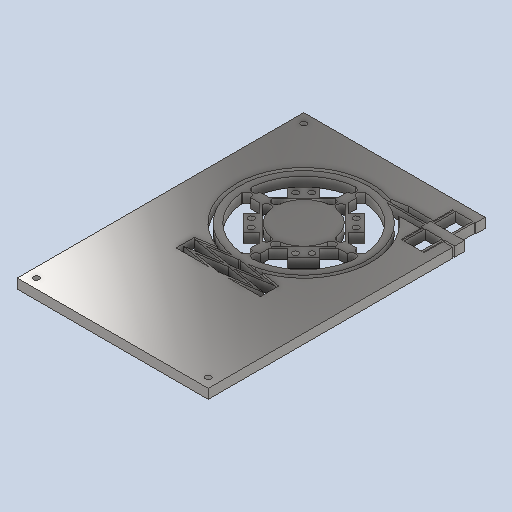
# Autodesk Inventor part: FlexBloc
Saved by Autodesk Inventor 2023 (Build 270158000, 158)
## iProperties
Created: 2023-03-17
Part Number: FlexBloc
Material: Steel, Mild
Document SubType Name: Modeling
Designer: Nathann
Density: 7.85 g/cm^3
Appearance: Semi-Polished
Mass: 505.648 g
Surface Area: 323.574 cm^2
Volume: 64.4137 cm^3
Author: Nathann
Autodesk Inventor part; units mm, degrees
ref_plane "YZ Plane" through (0, 0, 0) normal (1, 0, 0) x (0, 1, 0)
ref_plane "XZ Plane" through (0, 0, 0) normal (0, 1, 0) x (-1, 0, 0)
ref_plane "XY Plane" through (0, 0, 0) normal (0, 0, 1) x (1, 0, 0)
sketch "Sketch1" plane through (0, 0, 0) normal (0, 1, 0) x (-1, 0, 0)
  line L0 (0, 0) -> (100, 0)
  line L1 (100, 0) -> (100, 150)
  line L2 (100, 150) -> (0, 150)
  line L3 (0, 150) -> (0, 0)
  dimension "d0" = 150
  dimension "d1" = 100
  constraints: 8 end point, 2 parallel, 1 horizontal, 1 perpendicular
  measures "d0" distance of L2.end L0.start
  measures "d1" distance of L0.start L0.end
extrude "Extrusion1" add sketch "Sketch1" along normal blind 5
sketch "Sketch6" plane through (0, 5, 0) normal (0, 1, 0) x (1, 0, 0)
  circle A0 centre (-50, -50) radius 15
  line L0 (0, -150) -> (0, 0) projected
  line L1 (0, 0) -> (-100, 0) projected
  circle A1 centre (-50, -50) radius 30
  circle A2 centre (-50, -50) radius 33.541
  line L2 (-64.4545, -50.5) -> (-85.4944, -50.5)
  line L3 (-85.4944, -50.5) -> (-85.4944, -49.5)
  line L4 (-85.4944, -49.5) -> (-64.4545, -49.5)
  line L5 (-64.4545, -49.5) -> (-64.4545, -50.5)
  line L6 (-50, -50) -> (-59.276, -50)
  circle A3 centre (-50, -50) radius 36.041
  line L7 (-65, -50) -> (-80, -50)
  line L8 (-67.5, -50) -> (-70, -52.5)
  line L9 (-67.5, -50) -> (-70, -47.5)
  line L10 (-70, -52.5) -> (-70.7463, -51.7537)
  line L11 (-70, -47.5) -> (-74.2837, -51.7837)
  line L12 (-70, -52.5) -> (-72.5, -50)
  line L13 (-72.5, -50) -> (-70, -47.5)
  line L14 (-73.2071, -50) -> (-70.3536, -52.8536)
  line L15 (-70.3536, -52.8536) -> (-70, -52.5)
  line L16 (-73.2071, -50) -> (-70.3536, -47.1464)
  line L17 (-70.3536, -47.1464) -> (-70, -47.5)
  line L18 (-70.3536, -52.8536) -> (-65.8462, -57.3609)
  line L19 (-65.8462, -57.3609) -> (-65.1391, -56.6538)
  line L20 (-65.1391, -56.6538) -> (-69.6464, -52.1464)
  line L21 (-70.3536, -47.1464) -> (-65.8462, -42.6391)
  line L22 (-65.8462, -42.6391) -> (-65.1391, -43.3462)
  line L23 (-65.1391, -43.3462) -> (-69.6464, -47.8536)
  line L24 (-50, -50) -> (-54.8166, -54.8166)
  line L25 (-50, -50) -> (-57.7269, -42.2731)
  line L26 (-65.1391, -56.6538) -> (-70.0888, -61.6036)
  line L27 (-70.0888, -61.6036) -> (-65.8462, -65.8462)
  line L28 (-65.8462, -65.8462) -> (-60.8964, -60.8964)
  line L29 (-60.8964, -60.8964) -> (-65.1391, -56.6538)
  circle A4 centre (-65.8462, -61.6036) radius 1.5
  line L30 (-64.4545, -50) -> (-69.6304, -50)
  line L31 (-65.1391, -43.3462) -> (-70.0888, -38.3964)
  line L32 (-70.0888, -38.3964) -> (-65.8462, -34.1538)
  line L33 (-65.8462, -34.1538) -> (-60.8964, -39.1036)
  line L34 (-60.8964, -39.1036) -> (-65.1391, -43.3462)
  circle A5 centre (-65.8462, -38.3964) radius 1.5
  line L35 (-50, -64.4545) -> (-50, -69.6304)
  line L36 (-34.1538, -65.8462) -> (-39.1036, -60.8964)
  line L37 (-39.1036, -60.8964) -> (-43.3462, -65.1391)
  line L38 (-42.6391, -65.8462) -> (-43.3462, -65.1391)
  circle A6 centre (-38.3964, -65.8462) radius 1.5
  line L39 (-43.3462, -65.1391) -> (-38.3964, -70.0888)
  line L40 (-50, -67.5) -> (-52.5, -70)
  line L41 (-50, -67.5) -> (-47.5, -70)
  line L42 (-47.1464, -70.3536) -> (-42.6391, -65.8462)
  line L43 (-49.5, -64.4545) -> (-49.5, -85.4944)
  line L44 (-43.3462, -65.1391) -> (-47.8536, -69.6464)
  line L45 (-50.5, -85.4944) -> (-50.5, -64.4545)
  line L46 (-47.5, -70) -> (-48.2463, -70.7463)
  line L47 (-49.5, -85.4944) -> (-50.5, -85.4944)
  line L48 (-38.3964, -70.0888) -> (-34.1538, -65.8462)
  line L49 (-50.5, -64.4545) -> (-49.5, -64.4545)
  line L50 (-50, -65) -> (-50, -80)
  line L51 (-47.1464, -70.3536) -> (-47.5, -70)
  line L52 (-52.8536, -70.3536) -> (-52.5, -70)
  line L53 (-47.5, -70) -> (-50, -72.5)
  line L54 (-50, -73.2071) -> (-47.1464, -70.3536)
  line L55 (-50, -72.5) -> (-52.5, -70)
  line L56 (-50, -73.2071) -> (-52.8536, -70.3536)
  line L57 (-52.5, -70) -> (-48.2163, -74.2837)
  line L58 (-56.6538, -65.1391) -> (-52.1464, -69.6464)
  line L59 (-52.8536, -70.3536) -> (-57.3609, -65.8462)
  line L60 (-60.8964, -60.8964) -> (-56.6538, -65.1391)
  line L61 (-56.6538, -65.1391) -> (-61.6036, -70.0888)
  circle A7 centre (-61.6036, -65.8462) radius 1.5
  line L62 (-65.8462, -65.8462) -> (-60.8964, -60.8964)
  line L63 (-61.6036, -70.0888) -> (-65.8462, -65.8462)
  line L64 (-57.3609, -65.8462) -> (-56.6538, -65.1391)
  line L65 (-35.5455, -50) -> (-30.3696, -50)
  line L66 (-34.1538, -34.1538) -> (-39.1036, -39.1036)
  line L67 (-39.1036, -39.1036) -> (-34.8609, -43.3462)
  line L68 (-34.1538, -42.6391) -> (-34.8609, -43.3462)
  circle A8 centre (-34.1538, -38.3964) radius 1.5
  line L69 (-34.8609, -43.3462) -> (-29.9112, -38.3964)
  line L70 (-32.5, -50) -> (-30, -52.5)
  line L71 (-32.5, -50) -> (-30, -47.5)
  line L72 (-29.6464, -47.1464) -> (-34.1538, -42.6391)
  line L73 (-35.5455, -49.5) -> (-14.5056, -49.5)
  line L74 (-34.8609, -43.3462) -> (-30.3536, -47.8536)
  line L75 (-14.5056, -50.5) -> (-35.5455, -50.5)
  line L76 (-30, -47.5) -> (-29.2537, -48.2463)
  line L77 (-14.5056, -49.5) -> (-14.5056, -50.5)
  line L78 (-29.9112, -38.3964) -> (-34.1538, -34.1538)
  line L79 (-35.5455, -50.5) -> (-35.5455, -49.5)
  line L80 (-35, -50) -> (-20, -50)
  line L81 (-29.6464, -47.1464) -> (-30, -47.5)
  line L82 (-29.6464, -52.8536) -> (-30, -52.5)
  line L83 (-30, -47.5) -> (-27.5, -50)
  line L84 (-26.7929, -50) -> (-29.6464, -47.1464)
  line L85 (-27.5, -50) -> (-30, -52.5)
  line L86 (-26.7929, -50) -> (-29.6464, -52.8536)
  line L87 (-30, -52.5) -> (-25.7163, -48.2163)
  line L88 (-34.8609, -56.6538) -> (-30.3536, -52.1464)
  line L89 (-29.6464, -52.8536) -> (-34.1538, -57.3609)
  line L90 (-39.1036, -60.8964) -> (-34.8609, -56.6538)
  line L91 (-34.8609, -56.6538) -> (-29.9112, -61.6036)
  circle A9 centre (-34.1538, -61.6036) radius 1.5
  line L92 (-34.1538, -65.8462) -> (-39.1036, -60.8964)
  line L93 (-29.9112, -61.6036) -> (-34.1538, -65.8462)
  line L94 (-34.1538, -57.3609) -> (-34.8609, -56.6538)
  line L95 (-50, -35.5455) -> (-50, -30.3696)
  line L96 (-65.8462, -34.1538) -> (-60.8964, -39.1036)
  line L97 (-60.8964, -39.1036) -> (-56.6538, -34.8609)
  line L98 (-57.3609, -34.1538) -> (-56.6538, -34.8609)
  circle A10 centre (-61.6036, -34.1538) radius 1.5
  line L99 (-56.6538, -34.8609) -> (-61.6036, -29.9112)
  line L100 (-50, -32.5) -> (-47.5, -30)
  line L101 (-50, -32.5) -> (-52.5, -30)
  line L102 (-52.8536, -29.6464) -> (-57.3609, -34.1538)
  line L103 (-50.5, -35.5455) -> (-50.5, -14.5056)
  line L104 (-56.6538, -34.8609) -> (-52.1464, -30.3536)
  line L105 (-49.5, -14.5056) -> (-49.5, -35.5455)
  line L106 (-52.5, -30) -> (-51.7537, -29.2537)
  line L107 (-50.5, -14.5056) -> (-49.5, -14.5056)
  line L108 (-61.6036, -29.9112) -> (-65.8462, -34.1538)
  line L109 (-49.5, -35.5455) -> (-50.5, -35.5455)
  line L110 (-50, -35) -> (-50, -20)
  line L111 (-52.8536, -29.6464) -> (-52.5, -30)
  line L112 (-47.1464, -29.6464) -> (-47.5, -30)
  line L113 (-52.5, -30) -> (-50, -27.5)
  line L114 (-50, -26.7929) -> (-52.8536, -29.6464)
  line L115 (-50, -27.5) -> (-47.5, -30)
  line L116 (-50, -26.7929) -> (-47.1464, -29.6464)
  line L117 (-47.5, -30) -> (-51.7837, -25.7163)
  line L118 (-43.3462, -34.8609) -> (-47.8536, -30.3536)
  line L119 (-47.1464, -29.6464) -> (-42.6391, -34.1538)
  line L120 (-39.1036, -39.1036) -> (-43.3462, -34.8609)
  line L121 (-43.3462, -34.8609) -> (-38.3964, -29.9112)
  circle A11 centre (-38.3964, -34.1538) radius 1.5
  line L122 (-34.1538, -34.1538) -> (-39.1036, -39.1036)
  line L123 (-38.3964, -29.9112) -> (-34.1538, -34.1538)
  line L124 (-42.6391, -34.1538) -> (-43.3462, -34.8609)
  point P0 (-67.9675, -36.2751)
  point P1 (-63.7249, -67.9675)
  point P2 (-32.0325, -63.7249)
  point P3 (-36.2751, -32.0325)
  point P4 (-49.5, -72.7071)
  point P5 (-49.5, -79.9958)
  point P6 (-20.0042, -50.5)
  point P7 (-27.2929, -50.5)
  point P8 (-34.1538, -42.6391)
  point P9 (-27.2929, -49.5)
  point P10 (-20.0042, -49.5)
  point P11 (-49.5, -20.0042)
  point P12 (-49.5, -27.2929)
  point P13 (-68, -49.5)
  point P14 (-64.9917, -49.5)
  point P15 (-50.5, -35.0083)
  point P16 (-50.5, -32)
  point P17 (-49.5, -32)
  point P18 (-49.5, -35.0083)
  point P19 (-35.0083, -49.5)
  point P20 (-32, -49.5)
  point P21 (-32, -50.5)
  point P22 (-35.0083, -50.5)
  point P23 (-49.5, -64.9917)
  point P24 (-49.5, -68)
  point P25 (-50.5, -68)
  point P26 (-50.5, -64.9917)
  point P27 (-64.9917, -50.5)
  point P28 (-68, -50.5)
  point P29 (-57.3609, -34.1538)
  point P30 (-50.5, -27.2929)
  point P31 (-50.5, -20.0042)
  point P32 (-79.9958, -49.5)
  point P33 (-72.7071, -49.5)
  point P34 (-72.7071, -50.5)
  point P35 (-79.9958, -50.5)
  point P36 (-50.5, -79.9958)
  point P37 (-50.5, -72.7071)
  point P38 (-83.5373, -50.5)
  point P39 (-83.5373, -49.5)
  point P40 (-50.5, -16.4627)
  point P41 (-49.5, -16.4627)
  point P42 (-16.4627, -49.5)
  point P43 (-16.4627, -50.5)
  point P44 (-49.5, -83.5373)
  point P45 (-50.5, -83.5373)
  dimension "d80" = 30
  dimension "d81" = 60
  dimension "d78" = 50
  dimension "d79" = 50
  dimension "d82" = 67.082
  dimension "d83" = 0.5
  dimension "d84" = 0.5
  dimension "d91" = 72.082
  dimension "d92" = 5
  dimension "d93" = 2.5
  dimension "d94" = 2.5
  dimension "d95" = 45
  dimension "d96" = 45
  dimension "d97" = 0.5
  dimension "d98" = 0.5
  dimension "d99" = 0.5
  dimension "d100" = 45
  dimension "d101" = 45
  dimension "d102" = 6
  dimension "d103" = 7
  dimension "d104" = 3
  dimension "d105" = 3
  dimension "d106" = 3
  dimension "d107" = 3
  dimension "d108" = 7.5
  dimension "d109" = 3
  dimension "d110" = 6
  dimension "d111" = 7
  dimension "d112" = 3
  dimension "d113" = 3
  dimension "d114" = 3
  dimension "d117" = 360
  constraints: 246 end point, 20 point on line, 15 perpendicular, 10 centre point, 9 parallel, 3 coincident, 3 horizontal, 3 midpoint, 264 other
  measures "d78" distance from line of point (-50, -50) L0
  measures "d79" distance from line of L1 point (-50, -50)
  measures "d82" diameter of A2
  measures "d83" distance between parallel lines of L4 L6
  measures "d84" distance from line of point (-50, -50) L2
  measures "d91" diameter of A3
  measures "d92" distance of L8.start L12.end
  measures "d93" horizontal distance of L12.end L9.end
  measures "d94" horizontal distance of L8.end L12.end
  measures "d95" angle of L7 L8
  measures "d96" angle of L9 L7
  measures "d97" distance of L14.end L8.end
  measures "d98" distance between parallel lines of L10 L20
  measures "d99" distance between parallel lines of L23 L11
  measures "d100" angle of L24 L6
  measures "d101" angle of L25 L6
  measures "d102" distance of L28.end L19.end
  measures "d103" distance of L19.end L26.end
  measures "d104" distance from line of L27 A4.centre
  measures "d105" distance from line of L26 A4.centre
  measures "d106" diameter of A4
  measures "d107" distance from line of L24 A4.centre
  measures "d108" distance of L7.start L12.end
  measures "d109" distance of point (-67.968, -36.275) A5.centre
  measures "d110" distance of L33.end L22.end
  measures "d111" distance of L32.end L33.end
  measures "d112" distance from line of L33 A5.centre
  measures "d113" diameter of A5
  measures "d114" distance from line of A5.centre L25
extrude "Extrusion6" cut sketch "Sketch6" against normal blind 10 contours A0 L105 L100 L118 L120 L67 L74 L71 L73 | L75 L70 L88 L90 L37 L44 L41 L43 A0 | A0 L4 L9 L23 L34 L97 L104 L101 L103 | L84 L72 L69 L78 L123 L121 L119 L116 L105 A1 L73 | L45 L40 L58 L60 L29 L20 L8 L2 A0 | L75 A1 L43 L54 L42 L39 L48 L93 L91 L89 L86 | A2 L73 L77 L75 | L114 L102 L99 L108 L32 L31 L21 L16 L4 A1 L103 | A2 L103 L107 L105 | L45 A1 L2 L14 L18 L26 L27 L63 L61 L59 L56 | L43 L47 L45 A2 | A2 L2 L3 L4 | A4 | A5 | A6 | A7 | A8 | A9 | A10 | A11
sketch "Sketch7" plane through (0, 5, 0) normal (0, 1, 0) x (1, 0, 0)
  line L0 (-30.2515, -22) -> (6.5047, -22)
  line L1 (6.5047, -22) -> (6.5047, -15)
  line L2 (6.5047, -15) -> (-23.9617, -15)
  line L3 (-50, -60) -> (-28.7023, -38.7023)
  line L4 (-50, -60) -> (0, -60)
  line L5 (-11.682, -22) -> (-5.682, -22)
  line L6 (-2.365, -15) -> (-8.365, -15)
  line L7 (-5, -22) -> (-17, -22)
  line L8 (-17, -22) -> (-17, -32)
  line L9 (-17, -32) -> (-5, -32)
  line L10 (-5, -32) -> (-5, -22)
  line L11 (-5, -15) -> (-17, -15)
  line L12 (-17, -15) -> (-17, -5)
  line L13 (-17, -5) -> (-5, -5)
  line L14 (-5, -5) -> (-5, -15)
  line L15 (0, 0) -> (-100, 0) projected
  line L16 (0, -150) -> (0, 0) projected
  line L17 (-16.5, -32) -> (-15.5, -32)
  line L18 (-15.5, -32) -> (-15.5, -21)
  line L19 (-15.5, -21) -> (-16.5, -21)
  line L20 (-16.5, -21) -> (-16.5, -32)
  line L21 (-5.5, -32) -> (-6.5, -32)
  line L22 (-6.5, -32) -> (-6.5, -21)
  line L23 (-6.5, -21) -> (-5.5, -21)
  line L24 (-5.5, -21) -> (-5.5, -32)
  line L25 (-5.5, -5) -> (-6.5, -5)
  line L26 (-6.5, -5) -> (-6.5, -16)
  line L27 (-6.5, -16) -> (-5.5, -16)
  line L28 (-5.5, -16) -> (-5.5, -5)
  line L29 (-16.5, -5) -> (-15.5, -5)
  line L30 (-15.5, -5) -> (-15.5, -16)
  line L31 (-15.5, -16) -> (-16.5, -16)
  line L32 (-16.5, -16) -> (-16.5, -5)
  line L33 (-17.539, -21) -> (0, -21)
  line L34 (0, -21) -> (0, -16)
  line L35 (0, -16) -> (-17.539, -16)
  arc A0 (-49.5, -16.4627) -> (-50.5, -16.4627) centre (-50, -50) ccw projected
  line L36 (0, 0) -> (-5, 0)
  line L37 (-5, 0) -> (-5, -16)
  line L38 (-5, -16) -> (0, -16)
  line L39 (0, -16) -> (0, 0)
  line L40 (-17.539, -21) -> (-17.539, -16)
  line L41 (-20.9617, -19) -> (-17.539, -19)
  line L42 (-17.539, -19) -> (-17.539, -18)
  line L43 (-17.539, -18) -> (-20.9617, -18)
  line L44 (-23.9617, -15) -> (-23.9617, -22)
  line L45 (-23.9617, -22) -> (-30.2515, -22)
  line L46 (-20.9617, -18) -> (-20.9617, -19)
  point P0 (-5.5, -10.5)
  point P1 (-5, -27)
  point P2 (-16, -21)
  point P3 (-16, -16)
  point P4 (-17, -15)
  point P5 (-17, -22)
  point P6 (-15.5, -5)
  point P7 (-15.5, -16)
  point P8 (-6.5, -16)
  point P9 (-6.5, -5)
  point P10 (-5.5, -16)
  point P11 (0, -16)
  point P12 (0, -15)
  point P13 (0, -21)
  point P14 (0, -22)
  point P15 (-6.5, -32)
  point P16 (-5, -5)
  point P17 (-15.5, -15)
  point P18 (-16.5, -15)
  point P19 (-15.5, -22)
  point P20 (-16.5, -22)
  point P21 (-16.5, -15)
  point P22 (-16.5, -22)
  point P23 (-6.5, -22)
  point P24 (-15.5, -22)
  point P25 (-5.5, -22)
  point P26 (-5.5, -15)
  point P27 (-15.5, -15)
  point P28 (-6.5, -15)
  dimension "d125" = 45
  dimension "d128" = 10
  dimension "d133" = 12
  dimension "d134" = 12
  dimension "d135" = 5
  dimension "d136" = 1
  dimension "d137" = 1
  dimension "d138" = 1
  dimension "d139" = 1
  dimension "d140" = 0.5
  dimension "d141" = 0.5
  dimension "d142" = 11
  dimension "d144" = 11
  dimension "d145" = 11
  dimension "d146" = 10
  dimension "d147" = 11
  dimension "d164" = 5
  dimension "d169" = 0
  dimension "d170" = 5
  dimension "d171" = 1
  dimension "d172" = 2
  dimension "d202" = 5
  dimension "d214" = 3
  constraints: 90 end point, 17 parallel, 17 point on line, 13 horizontal, 12 perpendicular, 4 midpoint, 2 vertical
  measures "d125" angle of L3 L4
  measures "d128" distance of L9.end L7.start
  measures "d133" distance of L8.end L9.end
  measures "d134" distance of L12.end L13.end
  measures "d135" distance between parallel lines of L16 L10
  measures "d136" distance between parallel lines of L18 L20
  measures "d137" distance between parallel lines of L22 L24
  measures "d138" distance from line of L26 point (-5.5, -10.5)
  measures "d139" distance between parallel lines of L32 L30
  measures "d140" distance between parallel lines of L8 L20
  measures "d141" distance from line of point (-5, -27) L24
  measures "d142" distance of L17.end L18.end
  measures "d144" distance of L29.end L30.end
  measures "d145" distance of L27.end L25.start
  measures "d146" distance of L11.end L12.end
  measures "d147" distance of L21.end L22.end
  measures "d164" distance between parallel lines of L16 L37
  measures "d169" distance between parallel lines of L34 L16
  measures "d170" distance between parallel lines of L35 L33
  measures "d171" distance between parallel lines of L43 L41
  measures "d172" distance between parallel lines of L35 L43
  measures "d202" distance between parallel lines of L15 L13
  measures "d214" distance between parallel lines of L46 L44
extrude "Extrusion7" cut sketch "Sketch7" against normal blind 5 contours L44 L2 L32 L35 L40 L43 L46 L41 L33 L20 L0 | L0 L20 L9 L8 | L12 L13 L32 L2 | L18 L33 L22 L0 | L0 L22 L9 L18 | L30 L13 L26 L2 | L2 L26 L35 L30 | L24 L0 L10 L9 | L33 L16 L0 L24 | L16 L2 L1 L0 | L28 L13 L14 L2 | L2 L37 L35 L28 | L35 L37 L2 L16 | L14 L37 L15 L16 L2
sketch "Sketch9" plane through (0, 5, 0) normal (0, 1, 0) x (1, 0, 0)
  arc A0 (-35.0083, -49.5) -> (-49.5, -35.0083) centre (-50, -50) ccw projected
  line L0 (-50, -50) -> (-50, -7.3451)
  arc A1 (-49.5, -16.4627) -> (-50.5, -16.4627) centre (-50, -50) ccw projected
  line L1 (-50, -16.459) -> (-35, -13.959)
  line L2 (-35, -13.959) -> (-50, -11.459)
  line L3 (-50, -11.459) -> (-65, -13.959)
  line L4 (-65, -13.959) -> (-50, -16.459)
  line L5 (-50, -17.4728) -> (-28.9172, -13.959)
  line L6 (-28.9172, -13.959) -> (-50, -10.4452)
  line L7 (-50, -10.4452) -> (-71.0828, -13.959)
  line L8 (-71.0828, -13.959) -> (-50, -17.4728)
  line L9 (-28.9172, -13.959) -> (-71.0828, -13.959)
  line L10 (-65, -7.9452) -> (-50, -10.4452)
  line L11 (-71.0828, -7.9452) -> (-50, -11.459)
  line L12 (-50, -5.4452) -> (-65, -7.9452)
  line L13 (-50, -4.4314) -> (-71.0828, -7.9452)
  line L14 (-28.9172, -7.9452) -> (-71.0828, -7.9452)
  line L15 (-35, -7.9452) -> (-50, -5.4452)
  line L16 (-50, -11.459) -> (-28.9172, -7.9452)
  line L17 (-28.9172, -7.9452) -> (-50, -4.4314)
  line L18 (-50, -10.4452) -> (-35, -7.9452)
  arc A2 (-49.5, -16.4627) -> (-50.5, -16.4627) centre (-50, -50) ccw projected
  line L19 (-50, -50) -> (-50, -44.5788)
  line L20 (-57.3177, -17.267) -> (-72.0828, -14.8061)
  line L21 (-72.0828, -14.8061) -> (-72.0828, -5.2647)
  line L22 (-42.6823, -17.267) -> (-27.9172, -14.8061)
  line L23 (-27.9172, -14.8061) -> (-27.9172, -5.2647)
  line L24 (-23.9617, -15) -> (-17, -15) projected
  line L25 (-27.9172, -5.2647) -> (-45, -5.2647)
  line L26 (-55, -5.2647) -> (-72.0828, -5.2647)
  line L27 (-57.3177, -17.267) -> (-54.3685, -16.7447)
  line L28 (-42.6823, -17.267) -> (-45.6315, -16.7447)
  line L29 (-57.3177, -50) -> (-38.2747, -50)
  line L30 (-50, -83.541) -> (-35, -86.041)
  line L31 (-35, -86.041) -> (-50, -88.541)
  line L32 (-50, -88.541) -> (-65, -86.041)
  line L33 (-65, -86.041) -> (-50, -83.541)
  line L34 (-50, -82.5272) -> (-28.9172, -86.041)
  line L35 (-28.9172, -86.041) -> (-50, -89.5548)
  line L36 (-50, -89.5548) -> (-71.0828, -86.041)
  line L37 (-71.0828, -86.041) -> (-50, -82.5272)
  line L38 (-28.9172, -86.041) -> (-71.0828, -86.041)
  line L39 (-65, -92.0548) -> (-50, -89.5548)
  line L40 (-71.0828, -92.0548) -> (-50, -88.541)
  line L41 (-50, -94.5548) -> (-65, -92.0548)
  line L42 (-50, -95.5686) -> (-71.0828, -92.0548)
  line L43 (-28.9172, -92.0548) -> (-71.0828, -92.0548)
  line L44 (-35, -92.0548) -> (-50, -94.5548)
  line L45 (-50, -88.541) -> (-28.9172, -92.0548)
  line L46 (-28.9172, -92.0548) -> (-50, -95.5686)
  line L47 (-50, -89.5548) -> (-35, -92.0548)
  line L48 (-57.3177, -82.733) -> (-72.0828, -85.1939)
  line L49 (-72.0828, -85.1939) -> (-72.0828, -94.7353)
  line L50 (-42.6823, -82.733) -> (-27.9172, -85.1939)
  line L51 (-27.9172, -85.1939) -> (-27.9172, -94.7353)
  line L52 (-27.9172, -94.7353) -> (-45, -94.7353)
  line L53 (-55, -94.7353) -> (-72.0828, -94.7353)
  line L54 (-57.3177, -82.733) -> (-54.3685, -83.2553)
  line L55 (-42.6823, -82.733) -> (-45.6315, -83.2553)
  point P0 (0, 0)
  point P1 (-16.459, -50)
  point P2 (-16.459, -50)
  point P3 (-50, -1.3313)
  point P4 (-51, -4.2647)
  point P5 (-51, -4.5981)
  point P6 (-53.0414, -10.9521)
  point P7 (-46.9586, -10.9521)
  point P8 (-45.6315, -16.7447)
  point P9 (-51.4257, -26.4893)
  point P10 (-50, -26.459)
  point P11 (-42.6823, -17.267)
  point P12 (-57.3177, -17.267)
  point P13 (-49.5, -64.9917)
  point P14 (-50, -92.6549)
  point P15 (-50, -98.6687)
  point P16 (-51, -95.7353)
  point P17 (-51, -95.4019)
  point P18 (-51.4257, -73.5107)
  point P19 (-50, -73.541)
  point P20 (-50, -55.4212)
  point P21 (-23.9617, -85)
  point P22 (-49.5, -83.5373)
  point P23 (-50.5, -83.5373)
  point P24 (-53.0414, -89.0479)
  point P25 (-46.9586, -89.0479)
  dimension "d167" = 5
  dimension "d168" = 1
  dimension "d179" = 1
  dimension "d180" = 1
  dimension "d182" = 1.0138
  dimension "d185" = 6.0138
  dimension "d190" = 1
  dimension "d191" = 1
  dimension "d203" = 0
  dimension "d204" = 1
  dimension "d205" = 1
  dimension "d206" = 1
  dimension "d207" = 1
  dimension "d208" = 5
  dimension "d209" = 5
  constraints: 110 end point, 37 symmetric about line, 19 point on line, 5 equal length, 5 parallel, 4 horizontal, 3 vertical, 2 perpendicular, 34 other
  measures "d167" distance of L1.start L2.end
  measures "d168" distance between parallel lines of L5 L1
  measures "d179" distance between parallel lines of L8 L4
  measures "d180" distance between parallel lines of L7 L3
  measures "d182" distance of L5.start L1.start
  measures "d185" distance of L5.start L11.end
  measures "d190" horizontal distance of L13.start point (-51, -4.265)
  measures "d191" horizontal distance of point (-51, -4.598) L13.start
  measures "d203" distance between parallel lines of L19 L0
  measures "d204" distance between parallel lines of L8 L20
  measures "d205" distance between parallel lines of L5 L22
  measures "d206" distance from line of L5.end L23
  measures "d207" distance from line of L21 L7.end
  measures "d208" horizontal distance of L25.end L13.start
  measures "d209" horizontal distance of L13.start L26.start
extrude "Extrusion10" cut sketch "Sketch9" against normal blind 5 contours L30 L38 L33 | L31 L32 L38 | L34 L55 L50 L51 L52 L46 L45 L35 | L36 L40 L42 L53 L49 L48 L54 L37 | L47 L43 L39 | L43 L44 L41
sketch "Sketch11" plane through (0, 5, 0) normal (0, 1, 0) x (1, 0, 0)
  arc A0 (-64.9917, -50.5) -> (-50.5, -64.9917) centre (-50, -50) ccw projected
  circle A1 centre (-50, -50) radius 33.541
  line L0 (-49.5, -85.4944) -> (-49.5, -83.5373) projected
  arc A2 (-74.717, -75.4789) -> (-25.283, -75.4789) centre (-50, -50) ccw
  arc A3 (-15.5761, -58.6662) -> (-40.2932, -15.855) centre (-50, -50) ccw
  arc A4 (-59.7068, -15.855) -> (-84.8937, -56.5221) centre (-50, -50) ccw
  circle A5 centre (-50, -50) radius 35.498
  line L1 (-57.3177, -82.733) -> (-54.3685, -83.2553) projected
  line L2 (-57.3177, -82.733) -> (-61.7985, -83.4799)
  line L3 (-57.3177, -82.733) -> (-72.0828, -85.1939) projected
  line L4 (-27.9172, -85.1939) -> (-42.6823, -82.733) projected
  line L5 (-38.2015, -83.4799) -> (-42.6823, -82.733)
  point P0 (0, 0)
  point P1 (-82.0065, -60.0292)
  point P2 (-38.2015, -83.4799)
  point P3 (-25.283, -75.4789)
  point P4 (-40.2932, -15.855)
  point P5 (-59.7068, -15.855)
  dimension "d220" = 67.082
  constraints: 11 point on circle, 5 centre point, 4 end point, 3 coincident, 2 point on line, 1 collinear
  measures "d220" diameter of A1
extrude "Extrusion11" cut sketch "Sketch11" against normal blind 5 contours A1 L2 A2 A5 A4 A3 L4
sketch "Sketch12" plane through (0, 5, 0) normal (0, 1, 0) x (1, 0, 0)
  line L0 (-17, -15) -> (-23.9617, -15) projected
  line L1 (-23.9617, -15) -> (-30.0605, -15)
  line L2 (-30.0605, -15) -> (-30.0605, -22)
  line L3 (-30.0605, -22) -> (-23.9617, -22)
  line L4 (-23.9617, -22) -> (-23.9617, -15)
  line L5 (-30.0605, -22) -> (-38.2015, -16.5201)
  line L6 (-38.2015, -16.5201) -> (-30.0605, -15)
  point P0 (0, 0)
  constraints: 12 end point, 2 parallel, 1 horizontal, 1 perpendicular
extrude "Extrusion12" cut sketch "Sketch12" against normal blind 5
sketch "Sketch13" plane through (0, 5, 0) normal (0, 1, 0) x (1, 0, 0)
  line L0 (-17.539, -18) -> (-20.9617, -18) projected
  line L1 (-20.9617, -18) -> (-41.4723, -18)
  line L2 (-41.4723, -18) -> (-41.4723, -19)
  line L3 (-41.4723, -19) -> (-20.9617, -19)
  line L4 (-20.9617, -19) -> (-20.9617, -18)
  point P0 (0, 0)
  constraints: 8 end point, 2 parallel, 1 horizontal, 1 perpendicular
extrude "Extrusion13" add sketch "Sketch13" against normal blind 5
sketch "Sketch14" plane through (0, 5, 0) normal (0, 1, 0) x (1, 0, 0)
  circle A0 centre (-95, -5) radius 1.5
  circle A1 centre (-95, -145) radius 1.5
  circle A2 centre (-5, -145) radius 1.5
  line L0 (0, -150) -> (0, -22) projected
  line L1 (-100, -150) -> (0, -150) projected
  line L2 (-100, 0) -> (-100, -150) projected
  line L3 (-5, 0) -> (-100, 0) projected
  point P0 (0, 0)
  dimension "d227" = 5
  dimension "d228" = 5
  dimension "d229" = 5
  dimension "d230" = 5
  dimension "d231" = 5
  dimension "d232" = 5
  dimension "d233" = 3
  dimension "d234" = 3
  dimension "d235" = 3
  constraints: 3 centre point
  measures "d227" distance from line of L0 A2.centre
  measures "d228" distance from line of L1 A2.centre
  measures "d229" distance from line of L1 A1.centre
  measures "d230" distance from line of L2 A1.centre
  measures "d231" distance from line of L3 A0.centre
  measures "d232" distance from line of L2 A0.centre
  measures "d233" diameter of A0
  measures "d234" diameter of A1
  measures "d235" diameter of A2
extrude "Extrusion14" cut sketch "Sketch14" against normal blind 5
sketch "Sketch15" plane through (0, 5, 0) normal (0, 1, 0) x (1, 0, 0)
  line L0 (-47.5, -64.5161) -> (-52.5, -64.5161)
  line L1 (-52.5, -80.5042) -> (-47.5, -80.5042)
  arc A0 (-50.5, -35.0083) -> (-64.9917, -49.5) centre (-50, -50) ccw projected
  line L2 (-50, -50) -> (-45.827, -50)
  line L3 (-50.5, -72.7071) -> (-50.5, -79.9958) projected
  line L4 (-49.5, -68) -> (-49.5, -64.9917) projected
  circle A1 centre (-47.5, -77.5042) radius 2.15
  circle A2 centre (-52.5, -77.5042) radius 2.15
  line L5 (-50.5, -64.9917) -> (-50.5, -68) projected
  circle A3 centre (-52.5, -66.9902) radius 2.15
  circle A4 centre (-47.5, -66.9902) radius 2.15
  arc A5 (-79.9958, -50.5) -> (-50.5, -79.9958) centre (-50, -50) ccw projected
  line L6 (-50.5, -79.9958) -> (-49.5001, -80.0125)
  line L7 (-52.5, -64.7902) -> (-47.5, -64.7902)
  arc A6 (-49.5, -64.9917) -> (-35.0083, -50.5) centre (-50, -50) ccw projected
  line L8 (-52.5, -79.6542) -> (-52.5, -80.5042)
  line L9 (-47.5, -80.5042) -> (-47.5, -79.6542)
  line L10 (-47.5, -75.3542) -> (-47.5, -69.1402)
  line L11 (-47.5, -64.8402) -> (-47.5, -64.5161)
  line L12 (-52.5, -64.5161) -> (-52.5, -64.8402)
  line L13 (-52.5, -69.1402) -> (-52.5, -75.3542)
  circle A7 centre (-22.4958, -52.5) radius 2.15
  line L14 (-30.8598, -52.5) -> (-24.6458, -52.5)
  circle A8 centre (-33.0098, -52.5) radius 2.15
  line L15 (-35.4839, -47.5) -> (-35.4839, -52.5)
  line L16 (-35.1598, -47.5) -> (-35.4839, -47.5)
  line L17 (-35.4839, -52.5) -> (-35.1598, -52.5)
  circle A9 centre (-33.0098, -47.5) radius 2.15
  line L18 (-35.2098, -52.5) -> (-35.2098, -47.5)
  line L19 (-20.3458, -52.5) -> (-19.4958, -52.5)
  line L20 (-20.0042, -50.5) -> (-19.9875, -49.5001)
  line L21 (-24.6458, -47.5) -> (-30.8598, -47.5)
  line L22 (-19.4958, -52.5) -> (-19.4958, -47.5)
  line L23 (-19.4958, -47.5) -> (-20.3458, -47.5)
  circle A10 centre (-22.4958, -47.5) radius 2.15
  circle A11 centre (-47.5, -22.4958) radius 2.15
  line L24 (-47.5, -30.8598) -> (-47.5, -24.6458)
  circle A12 centre (-47.5, -33.0098) radius 2.15
  line L25 (-52.5, -35.4839) -> (-47.5, -35.4839)
  line L26 (-52.5, -35.1598) -> (-52.5, -35.4839)
  line L27 (-47.5, -35.4839) -> (-47.5, -35.1598)
  circle A13 centre (-52.5, -33.0098) radius 2.15
  line L28 (-47.5, -35.2098) -> (-52.5, -35.2098)
  line L29 (-47.5, -20.3458) -> (-47.5, -19.4958)
  line L30 (-49.5, -20.0042) -> (-50.4999, -19.9875)
  line L31 (-52.5, -24.6458) -> (-52.5, -30.8598)
  line L32 (-47.5, -19.4958) -> (-52.5, -19.4958)
  line L33 (-52.5, -19.4958) -> (-52.5, -20.3458)
  circle A14 centre (-52.5, -22.4958) radius 2.15
  circle A15 centre (-77.5042, -47.5) radius 2.15
  line L34 (-69.1402, -47.5) -> (-75.3542, -47.5)
  circle A16 centre (-66.9902, -47.5) radius 2.15
  line L35 (-64.5161, -52.5) -> (-64.5161, -47.5)
  line L36 (-64.8402, -52.5) -> (-64.5161, -52.5)
  line L37 (-64.5161, -47.5) -> (-64.8402, -47.5)
  circle A17 centre (-66.9902, -52.5) radius 2.15
  line L38 (-64.7902, -47.5) -> (-64.7902, -52.5)
  line L39 (-79.6542, -47.5) -> (-80.5042, -47.5)
  line L40 (-79.9958, -49.5) -> (-80.0125, -50.4999)
  line L41 (-75.3542, -52.5) -> (-69.1402, -52.5)
  line L42 (-80.5042, -47.5) -> (-80.5042, -52.5)
  line L43 (-80.5042, -52.5) -> (-79.6542, -52.5)
  circle A18 centre (-77.5042, -52.5) radius 2.15
  point P0 (0, 0)
  point P1 (-50.5, -66.4958)
  point P2 (-50, -80.5042)
  point P3 (-50.0001, -80.0042)
  point P4 (-33.5042, -50.5)
  point P5 (-19.9958, -50.0001)
  point P6 (-19.4958, -50)
  point P7 (-49.5, -33.5042)
  point P8 (-49.9999, -19.9958)
  point P9 (-50, -19.4958)
  point P10 (-66.4958, -49.5)
  point P11 (-80.0042, -49.9999)
  point P12 (-80.5042, -50)
  point P13 (-49.5, -66.2012)
  dimension "d238" = 2
  dimension "d240" = 0.7
  dimension "d241" = 4.3
  dimension "d243" = 1
  dimension "d244" = 3
  dimension "d245" = 3
  dimension "d246" = 0.5
  dimension "d247" = 4.3
  dimension "d248" = 4.3
  dimension "d249" = 2.2
  dimension "d250" = 2.2
  dimension "d253" = 360
  constraints: 82 end point, 33 point on circle, 16 centre point, 10 parallel, 8 point on line, 3 midpoint, 3 perpendicular, 2 horizontal, 1 tangent, 149 other
  measures "d241" diameter of A2
  measures "d243" distance from line of L4 point (-50.5, -66.496)
  measures "d244" vertical distance of point (-50, -80.504) A2.centre
  measures "d245" vertical distance of point (-50, -80.504) A1.centre
  measures "d246" distance of point (-50, -80.504) point (-50, -80.004)
  measures "d247" diameter of A3
  measures "d248" diameter of A4
  measures "d249" distance from line of L7 A3.centre
  measures "d250" distance from line of L7 A4.centre
extrude "Extrusion15" add sketch "Sketch15" against normal blind 5 contours L18 L16 A9 L21 A10 L23 L22 L19 A7 L14 A8 L17 | L26 A13 L31 A14 L33 L32 L29 A11 L24 A12 L27 L28 | L43 L42 L39 A15 L34 A16 L37 L38 L36 A17 L41 A18 | A6 L4 A4 L10 A1 L9 L1 L8 A5 L3 A2 L13 A3 L12 L7 | L11 A4 L4 A6 | A2 L3 A5 L8
sketch "Sketch16" plane through (0, 5, 0) normal (0, 1, 0) x (1, 0, 0)
  arc A0 (-52.5, -79.6542) -> (-50.5, -78.2932) centre (-52.5, -77.5042) ccw projected
  arc A1 (-47.5, -75.3542) -> (-49.5, -76.7152) centre (-47.5, -77.5042) ccw projected
  arc A2 (-48.7892, -68.7108) -> (-47.5, -69.1402) centre (-47.5, -66.9902) ccw projected
  arc A3 (-52.5, -69.1402) -> (-51.2108, -68.7108) centre (-52.5, -66.9902) ccw projected
  circle A4 centre (-52.5, -77.5042) radius 2.15
  circle A5 centre (-47.5, -77.5042) radius 2.15
  circle A6 centre (-47.5, -66.9902) radius 2.15
  circle A7 centre (-52.5, -66.9902) radius 2.15
  arc A8 (-50.5, -76.7152) -> (-52.5, -75.3542) centre (-52.5, -77.5042) ccw projected
  line L0 (-52.5, -75.3542) -> (-52.5, -79.6542)
  line L1 (-47.5, -79.8957) -> (-47.5, -79.6542) projected
  line L2 (-47.5, -79.6542) -> (-47.5, -75.3542)
  line L3 (-47.5, -69.2929) -> (-30.7071, -52.5) projected
  line L4 (-47.5, -69.2929) -> (-47.5, -64.8402)
  line L5 (-52.5, -69.1402) -> (-52.5, -64.8402)
  arc A9 (-64.7902, -52.5) -> (-52.5, -64.7902) centre (-50, -50) ccw projected
  line L6 (-30.8598, -52.5) -> (-35.1598, -52.5)
  line L7 (-30.7071, -47.5) -> (-35.1598, -47.5)
  circle A10 centre (-33.0098, -52.5) radius 2.15
  circle A11 centre (-33.0098, -47.5) radius 2.15
  circle A12 centre (-22.4958, -52.5) radius 2.15
  line L8 (-24.6458, -52.5) -> (-20.3458, -52.5)
  line L9 (-20.3458, -47.5) -> (-24.6458, -47.5)
  circle A13 centre (-22.4958, -47.5) radius 2.15
  line L10 (-47.5, -30.8598) -> (-47.5, -35.1598)
  line L11 (-52.5, -30.7071) -> (-52.5, -35.1598)
  circle A14 centre (-47.5, -33.0098) radius 2.15
  circle A15 centre (-52.5, -33.0098) radius 2.15
  circle A16 centre (-47.5, -22.4958) radius 2.15
  line L12 (-47.5, -24.6458) -> (-47.5, -20.3458)
  line L13 (-52.5, -20.3458) -> (-52.5, -24.6458)
  circle A17 centre (-52.5, -22.4958) radius 2.15
  line L14 (-69.1402, -47.5) -> (-64.8402, -47.5)
  line L15 (-69.2929, -52.5) -> (-64.8402, -52.5)
  circle A18 centre (-66.9902, -47.5) radius 2.15
  circle A19 centre (-66.9902, -52.5) radius 2.15
  circle A20 centre (-77.5042, -47.5) radius 2.15
  line L16 (-75.3542, -47.5) -> (-79.6542, -47.5)
  line L17 (-79.6542, -52.5) -> (-75.3542, -52.5)
  circle A21 centre (-77.5042, -52.5) radius 2.15
  point P0 (0, 0)
  point P1 (-23.2848, -50.5)
  point P2 (-49.5, -23.2848)
  point P3 (-76.7152, -49.5)
  point P4 (-52.5, -30.8598)
  point P5 (-30.8598, -47.5)
  point P6 (-69.1402, -52.5)
  point P7 (-47.5, -69.1402)
  dimension "d259" = 360
  constraints: 32 end point, 4 centre point, 4 coincident, 1 collinear, 1 concentric, 1 point on circle, 1 vertical, 118 other
extrude "Extrusion16" cut sketch "Sketch16" against normal blind 5 contours L0 A4 A0 | A4 L0 | L2 A5 A1 | A5 L2 | A6 L4 A2 | A10 L6 | L5 A7 A3 | A11 L7 | L8 A12 | A13 L9 | L10 A14 | A15 L11 | L12 A16 | A17 L13 | L14 A18 | A19 L15 | A20 L16 | A21 L17 picked at (-32.7557, -48.1701) picked at (-22.2208, -51.6584) picked at (-22.2417, -48.1701) picked at (-48.1701, -33.2639) picked at (-51.5827, -33.6231) picked at (-48.2613, -22.8821) picked at (-51.4469, -23.1945) picked at (-66.7361, -48.1701) picked at (-66.7361, -51.8299) picked at (-77.5906, -48.2114) picked at (-77.2501, -51.8299)
equation "\"d2\" = woodThickness"
equation "\"d83\" = 0.5 * bladeThickness"
equation "\"d84\" = 0.5 * bladeThickness"
equation "\"d93\" = 0.5 * d92"
equation "\"d94\" = d93"
equation "\"d97\" = 0.5 * bladeThickness"
equation "\"d98\" = d97"
equation "\"d99\" = d98"
equation "\"d104\" = 0.5 * d102"
equation "\"d105\" = d104"
equation "\"d106\" = M3Hole"
equation "\"d107\" = d102 - d105"
equation "\"d109\" = d104"
equation "\"d110\" = d102"
equation "\"d111\" = d103"
equation "\"d112\" = d107"
equation "\"d113\" = d106"
equation "\"d114\" = d107"
equation "\"bladeThickness\" = 1"
equation "\"woodThickness\" = 5"
equation "\"bladeLenghtFlexRatio\" = 0.05"
equation "\"colRadius\" = 3"
equation "\"d14\" = bladeThickness"
equation "\"d16\" = d14"
equation "\"d19\" = d16"
equation "\"M3Hole\" = 3"
body "Solid1"
